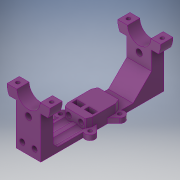
# Autodesk Inventor part: 000.401 - Держатель 1-ого звена
Saved by Autodesk Inventor 2019 (Build 230136000, 136)
## iProperties
Created: 2020-02-28
Part Number: 000.401 - Держатель 1-ого звена
Material: Пластик АБС
Document SubType Name: Modeling
Designer: Петров Иван
Density: 1.06 g/cm^3
Appearance: Гладкий — пурпурный
Author: Петров Иван
Autodesk Inventor part; units mm, degrees
ref_plane "YZ Plane" through (0, 0, 0) normal (1, 0, 0) x (0, 1, 0)
ref_plane "XZ Plane" through (0, 0, 0) normal (0, 1, 0) x (-1, 0, 0)
ref_plane "XY Plane" through (0, 0, 0) normal (0, 0, 1) x (1, 0, 0)
sketch "Эскиз1" plane through (0, 0, 0) normal (0, 1, 0) x (-1, 0, 0)
  line L0 (0, 0) -> (12.0208, -12.0208)
  line L1 (0, 0) -> (17, 0) construction
  circle A0 centre (12.0208, -12.0208) radius 1.5
  line L2 (0, 0) -> (12.0208, -12.0208) construction
  line L3 (-2.8284, -2.8284) -> (9.1924, -14.8492)
  line L4 (14.8492, -9.1924) -> (2.8284, 2.8284)
  arc A1 (2.8284, 2.8284) -> (-2.8284, -2.8284) centre (0, 0) ccw
  arc A2 (9.1924, -14.8492) -> (14.8492, -9.1924) centre (12.0208, -12.0208) ccw
  point P0 (6.0104, -6.0104)
  dimension "d0" = 17
  dimension "d1" = 45
  dimension "d2" = 3
  dimension "d3" = 8
  constraints: 12 end point, 4 point on circle, 4 tangent, 3 centre point, 3 equal length, 1 coincident, 1 horizontal, 1 midpoint
  measures "d0" distance of L0.start L0.end
  measures "d1" angle of L0 L1
  measures "d2" diameter of A0
  measures "d3" diameter of A2
extrude "Выдавливание1" add sketch "Эскиз1" along normal blind 4
pattern_circular "Круговой массив1" count 4 over 360 about axis through (0, 0, 0) along (0, 1, 0) of "Выдавливание1"
sketch "Эскиз2" plane through (0, 4, 0) normal (0, 1, 0) x (1, 0, 0)
  arc A0 (-14.8492, -9.1924) -> (-9.1924, -14.8492) centre (-12.0208, -12.0208) ccw projected
  arc A1 (14.8492, 9.1924) -> (9.1924, 14.8492) centre (12.0208, 12.0208) ccw projected
  line L0 (-9.1924, -14.8492) -> (9.1924, -14.8492)
  line L1 (9.1924, -14.8492) -> (9.1924, 14.8492)
  line L2 (9.1924, 14.8492) -> (-9.1924, 14.8492)
  line L3 (-9.1924, 14.8492) -> (-9.1924, -14.8492)
  point P0 (0, 0)
  constraints: 8 end point, 2 parallel, 1 perpendicular
extrude "Выдавливание2" add sketch "Эскиз2" against normal blind 4
sketch "Эскиз3" plane through (0, 4, 0) normal (0, 1, 0) x (1, 0, 0)
  line L0 (10, -12.2488) -> (-10, -12.2488)
  line L1 (-10, -12.2488) -> (-10, 14.8492)
  line L2 (-10, 14.8492) -> (10, 14.8492)
  line L3 (10, 14.8492) -> (10, -12.2488)
  line L4 (9.1924, 14.8492) -> (-9.1924, 14.8492) projected
  point P0 (0, 0)
  dimension "d11" = 20
  dimension "d12" = 27.098
  dimension "d17" = 0
  constraints: 8 end point, 2 parallel, 1 horizontal, 1 perpendicular
  measures "d11" distance of L1.end L2.end
  measures "d12" distance between parallel lines of L0 L2
  measures "d17" distance between parallel lines of L4 L2
extrude "Выдавливание3" add sketch "Эскиз3" along normal blind 7 and the other way blind 4
sketch "Эскиз4" plane through (-10, 4, 12.2488) normal (0, 0, 1) x (1, 0, 0)
  line L0 (13.75, 54.7) -> (10.5, 54.7)
  line L1 (10.5, 54.7) -> (10.5, 47.7)
  line L2 (10.5, 47.7) -> (20, 47.7)
  line L3 (20, 47.7) -> (20, 53.7)
  arc A0 (20, 53.7) -> (19, 54.7) centre (19, 53.7) ccw
  line L4 (19, 54.7) -> (16.15, 54.7)
  line L5 (16.15, 54.7) -> (16.15, 53.634)
  arc A1 (13.75, 53.634) -> (16.15, 53.634) centre (14.95, 51.85) ccw
  line L6 (13.75, 53.634) -> (13.75, 54.7)
  line L7 (9.5, 54.7) -> (9.5, 47.7)
  line L8 (9.5, 54.7) -> (6.25, 54.7)
  line L9 (6.25, 54.7) -> (6.25, 53.634)
  arc A2 (3.85, 53.634) -> (6.25, 53.634) centre (5.05, 51.85) ccw
  line L10 (3.85, 53.634) -> (3.85, 54.7)
  line L11 (3.85, 54.7) -> (1, 54.7)
  arc A3 (1, 54.7) -> (0, 53.7) centre (1, 53.7) ccw
  line L12 (0, 53.7) -> (0, 47.7)
  line L13 (0, 47.7) -> (9.5, 47.7)
  line L14 (9.5, 7) -> (9.5, 0)
  line L15 (0, 7) -> (9.5, 7)
  line L16 (0, 1) -> (0, 7)
  arc A4 (0, 1) -> (1, 0) centre (1, 1) ccw
  line L17 (3.85, 0) -> (1, 0)
  line L18 (3.85, 1.066) -> (3.85, 0)
  arc A5 (6.25, 1.066) -> (3.85, 1.066) centre (5.05, 2.85) ccw
  line L19 (6.25, 0) -> (6.25, 1.066)
  line L20 (9.5, 0) -> (6.25, 0)
  line L21 (10.5, 7) -> (20, 7)
  line L22 (10.5, 7) -> (10.5, 0)
  line L23 (13.75, 0) -> (10.5, 0)
  line L24 (13.75, 1.066) -> (13.75, 0)
  arc A6 (16.15, 1.066) -> (13.75, 1.066) centre (14.95, 2.85) ccw
  line L25 (16.15, 0) -> (16.15, 1.066)
  line L26 (19, 0) -> (16.15, 0)
  arc A7 (19, 0) -> (20, 1) centre (19, 1) ccw
  line L27 (20, 7) -> (20, 1)
  line L28 (20, 47.7) -> (20, 17)
  line L29 (20, 17) -> (20, 7)
  line L30 (0, 17) -> (0, 7)
  line L31 (0, 47.7) -> (0, 17)
  circle A8 centre (10, 17) radius 6.5
  circle A9 centre (10, 17) radius 5.4
  circle A10 centre (10, 17) radius 3.4957
  circle A11 centre (10, 17) radius 3.4957
  circle A12 centre (14.95, 51.85) radius 2.15
  circle A13 centre (5.05, 51.85) radius 2.15
  arc A14 (16.15, 1.066) -> (13.75, 1.066) centre (14.95, 2.85) ccw
  circle A15 centre (14.95, 2.85) radius 2.15
  circle A16 centre (5.05, 2.85) radius 2.15
  line L32 (13.75, 54.7) -> (10.5, 54.7)
  line L33 (16.15, 54.7) -> (13.75, 54.7)
  line L34 (13.75, 54.7) -> (6.25, 54.7)
  line L35 (6.25, 54.7) -> (3.85, 54.7)
  line L36 (16.15, 0) -> (13.75, 0)
  line L37 (6.25, 0) -> (6.25, 1.066)
  line L38 (6.25, 0) -> (3.85, 0)
  line L39 (9.5, 0) -> (10.5, 0)
  line L40 (10, 0) -> (10, -4)
  point P0 (10, -4)
  point P1 (0, 27.35)
  dimension "d18" = 4
  constraints: 82 end point, 18 point on circle, 15 centre point, 4 coincident, 2 concentric, 1 collinear, 1 horizontal, 1 midpoint, 1 perpendicular, 1 vertical, 6 other
  measures "d18" distance of L40.start L40.end
extrude "Выдавливание4" cut sketch "Эскиз4" against normal blind 10 contours A6 A15 | A16 A5
sketch "Эскиз5" plane through (0, 11, 0) normal (0, 1, 0) x (1, 0, 0)
  line L0 (-2.8, -2.2488) -> (-7.1, -2.2488) projected
  line L1 (-4.95, -2.2488) -> (-4.95, -4.2488)
  line L2 (-8.45, -6.2488) -> (-1.45, -6.2488)
  line L3 (-1.45, -6.2488) -> (-1.45, -2.2488)
  line L4 (-1.45, -2.2488) -> (-8.45, -2.2488)
  line L5 (-8.45, -2.2488) -> (-8.45, -6.2488)
  line L6 (-8.45, -6.2488) -> (-1.45, -2.2488) construction
  line L7 (-1.45, -6.2488) -> (-8.45, -2.2488) construction
  point P0 (0, 0)
  dimension "d21" = 2
  dimension "d22" = 7
  dimension "d23" = 4
  constraints: 14 end point, 3 midpoint, 2 parallel, 1 horizontal, 1 perpendicular, 1 vertical
  measures "d21" distance of L1.start L1.end
  measures "d22" distance of L4.end L3.end
  measures "d23" distance of L3.end L2.end
extrude "Выдавливание5" cut sketch "Эскиз5" against normal blind 17.5
mirror "Зеркальное отражение1" about plane through (0, 0, 0) normal (1, 0, 0) of "Выдавливание5"
sketch "Эскиз6" plane through (0, 0, 0) normal (0, -1, 0) x (1, 0, 0)
  line L0 (-10, 50) -> (10, 50)
  line L1 (10, 50) -> (10, -50)
  line L2 (10, -50) -> (-10, -50)
  line L3 (-10, -50) -> (-10, 50)
  line L4 (-10, 50) -> (10, -50) construction
  line L5 (10, 50) -> (-10, -50) construction
  point P0 (0, 0)
  dimension "d26" = 20
  dimension "d27" = 100
  constraints: 12 end point, 2 midpoint, 2 parallel, 1 horizontal, 1 perpendicular
  measures "d26" distance of L1.end L2.end
  measures "d27" distance of L0.end L1.end
extrude "Выдавливание6" add sketch "Эскиз6" against normal blind 4
chamfer "Фаска1" distance 2 angle 45 4 edges at (10, 7.5, 12.2488) (-10, 7.5, 12.2488) (10, 7.5, -14.8492) (-10, 7.5, -14.8492)
chamfer "Фаска2" distance 2 angle 45 4 edges at (10, 7.5, 10.2488) (-10, 7.5, 10.2488) (-10, 7.5, -12.8492) (10, 7.5, -12.8492)
sketch "Эскиз7" plane through (0, 4, 0) normal (0, 1, 0) x (1, 0, 0)
  line L0 (-10, -50) -> (10, -50) projected
  line L1 (10, -50) -> (10, -15.4728) projected
  line L2 (-10, -50) -> (10, -50)
  line L3 (10, -50) -> (10, -40)
  line L4 (10, -40) -> (-10, -40)
  line L5 (-10, -40) -> (-10, -50)
  line L6 (10, 50) -> (-10, 50) projected
  line L7 (-10, 50) -> (10, 50)
  line L8 (10, 50) -> (10, 40)
  line L9 (10, 40) -> (-10, 40)
  line L10 (-10, 40) -> (-10, 50)
  point P0 (0, 0)
  dimension "d36" = 10
  dimension "d37" = 20
  dimension "d38" = 10
  constraints: 16 end point, 4 parallel, 2 horizontal, 2 perpendicular, 1 point on line
  measures "d36" distance of L3.end L2.end
  measures "d37" distance of L8.end L9.end
  measures "d38" distance of L7.end L8.end
extrude "Выдавливание7" add sketch "Эскиз7" along normal blind 50 contours L5 L4 L1 L0
sketch "Эскиз8" plane through (-10, 0, 50) normal (0, 0, 1) x (1, 0, 0)
  line L0 (18, 4) -> (2, 4) projected
  line L1 (10, 4) -> (10, 41.7)
  circle A0 centre (10, 41.7) radius 9.5
  point P0 (10, 0)
  dimension "d41" = 37.7
  dimension "d42" = 19
  constraints: 2 end point, 1 centre point, 1 coincident, 1 midpoint, 1 vertical
  measures "d41" distance of L1.start L1.end
  measures "d42" diameter of A0
extrude "Выдавливание8" cut sketch "Эскиз8" against normal blind 133.25
sketch "Эскиз11" plane through (-10, 0, 50) normal (0, 0, 1) x (1, 0, 0)
  circle A0 centre (10, 41.7) radius 17.5
  circle A1 centre (10, 41.7) radius 9.5
  point P0 (10, 0)
  dimension "d49" = 35
  dimension "d78" = 19
  constraints: 2 centre point, 2 coincident
  measures "d49" diameter of A0
  measures "d78" diameter of A1
extrude "Выдавливание11" add sketch "Эскиз11" against normal blind 10
sketch "Эскиз12" plane through (0, 0, 0) normal (0, -1, 0) x (1, 0, 0)
  line L0 (-17.5, 40) -> (17.5, 40) projected
  line L1 (-10, 50) -> (10, 50) projected
  line L2 (17.5, 40) -> (10, 40)
  line L3 (10, 40) -> (10, 50)
  line L4 (10, 50) -> (17.5, 50)
  line L5 (17.5, 50) -> (17.5, 40)
  line L6 (10, 45) -> (17.5, 45)
  line L7 (17.5, 50) -> (17.5, 40) projected
  circle A0 centre (13.75, 45) radius 1.5
  line L8 (-17.5, 50) -> (-17.5, 40) projected
  line L9 (-10, 40) -> (-17.5, 40)
  line L10 (-17.5, 40) -> (-17.5, 50)
  line L11 (-17.5, 50) -> (-10, 50)
  line L12 (-10, 50) -> (-10, 40)
  line L13 (-10, 15.4728) -> (-10, 50) projected
  line L14 (-10, 45) -> (-17.5, 45)
  circle A1 centre (-13.75, 45) radius 1.5
  point P0 (0, 0)
  point P1 (10, 40)
  dimension "d52" = 3
  dimension "d53" = 3
  constraints: 20 end point, 5 midpoint, 4 parallel, 2 centre point, 2 horizontal, 2 perpendicular, 2 point on line
  measures "d52" diameter of A0
  measures "d53" diameter of A1
extrude "Выдавливание12" cut sketch "Эскиз12" against normal blind 57 contours A1 L14 | L14 A1 | A0 L6 | L6 A0
sketch "Эскиз13" plane through (0, 0, 0) normal (0, -1, 0) x (1, 0, 0)
  line L0 (-17.5, 40) -> (17.5, 40)
  line L1 (-10, 50) -> (10, 50)
  line L2 (17.5, 40) -> (10, 40)
  line L3 (10, 40) -> (10, 50)
  line L4 (10, 50) -> (17.5, 50)
  line L5 (17.5, 50) -> (17.5, 40)
  line L6 (10, 45) -> (17.5, 45)
  line L7 (17.5, 50) -> (17.5, 40)
  circle A0 centre (13.75, 45) radius 1.5
  line L8 (-17.5, 50) -> (-17.5, 40)
  line L9 (-10, 40) -> (-17.5, 40)
  line L10 (-17.5, 40) -> (-17.5, 50)
  line L11 (-17.5, 50) -> (-10, 50)
  line L12 (-10, 50) -> (-10, 40)
  line L13 (-10, 15.4728) -> (-10, 50)
  line L14 (-10, 45) -> (-17.5, 45)
  circle A1 centre (-13.75, 45) radius 1.5
  point P0 (0, 0)
  point P1 (0, 0)
  point P2 (10, 40)
  dimension "d56" = 3
  dimension "d57" = 3
  constraints: 30 end point, 5 midpoint, 4 parallel, 2 centre point, 2 horizontal, 2 perpendicular, 2 point on line
  measures "d56" diameter of A0
  measures "d57" diameter of A1
extrude "Выдавливание13" cut sketch "Эскиз13" against normal blind 34 contours L3 L6 A0 L5 L0 | L3 L4 L5 L6 A0 | A0 L6 | L6 A0
mirror "Зеркальное отражение2" about plane through (0, 0, 0) normal (1, 0, 0) of "Выдавливание13"
sketch "Эскиз14" plane through (-10, 0, 50) normal (0, 0, 1) x (1, 0, 0)
  circle A0 centre (10, 41.7) radius 9.5 projected
  line L0 (10, 41.7) -> (27.5, 41.7)
  arc A1 (25.715, 34) -> (-5.715, 34) centre (10, 41.7) ccw projected
  line L1 (10, 41.7) -> (-7.5, 41.7)
  point P0 (10, 0)
  constraints: 4 end point, 2 point on circle, 1 horizontal, 1 point on line
extrude "Выдавливание14" cut sketch "Эскиз14" against normal blind 35 contours L0 L1 A0 | A0 L1 A1 L0 picked at (3.7587, 42.4578)
mirror "Зеркальное отражение3" about plane through (0, 0, 0) normal (0, 0, 1) of "Выдавливание14", "Выдавливание12", "Выдавливание11", "Выдавливание7", "Выдавливание8", "Выдавливание13", "Зеркальное отражение2"
sketch "Эскиз15" plane through (-10, 0, 50) normal (0, 0, 1) x (1, 0, 0)
  circle A0 centre (5.05, 6.85) radius 2.15 projected
  circle A1 centre (14.95, 6.85) radius 2.15 projected
  point P0 (10, 0)
extrude "Выдавливание15" cut sketch "Эскиз15" against normal blind 10
sketch "Эскиз16" plane through (10, 4, 40) normal (0, 0, -1) x (-1, 0, 0)
  circle A0 centre (5.05, 2.85) radius 2.15 projected
  circle A1 centre (5.05, 2.85) radius 4.25
  circle A2 centre (14.95, 2.85) radius 2.15 projected
  circle A3 centre (14.95, 2.85) radius 4.25
  point P0 (10, -4)
  dimension "d64" = 8.5
  dimension "d65" = 8.5
  constraints: 2 centre point, 2 coincident
  measures "d64" diameter of A1
  measures "d65" diameter of A3
extrude "Выдавливание16" cut sketch "Эскиз16" along normal up to surface (27.7512 mm away)
chamfer "Фаска3" distance 3.75 angle 45 3 edges at (-9.0514, 4, 40) (0, 4, 40) (9.0514, 4, 40)
chamfer "Фаска4" distance 15 angle 45 1 edges at (0, 4, -40)
sketch "Эскиз17" plane through (-10, 0, 50) normal (0, 0, 1) x (1, 0, 0)
  arc A0 (0.5, 41.7) -> (19.5, 41.7) centre (10, 41.7) ccw projected
  line L0 (10, 32.2) -> (10, 27.2)
  circle A1 centre (10, 27.2) radius 2.6
  point P0 (10, 0)
  dimension "d74" = 5
  dimension "d75" = 5.2
  constraints: 2 end point, 1 centre point, 1 coincident, 1 point on circle, 1 vertical
  measures "d74" distance of L0.start L0.end
  measures "d75" diameter of A1
extrude "Выдавливание17" cut sketch "Эскиз17" against normal blind 143.75
equation "\"d36\" = d38"
